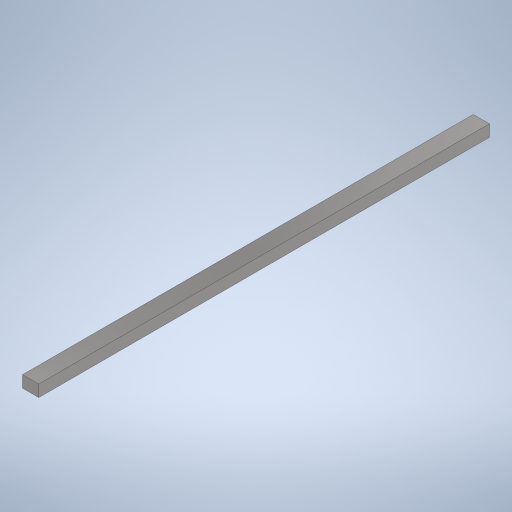
# Autodesk Inventor part: MGN9_rail
Saved by Autodesk Inventor 2024 (Build 280153000, 153)
## iProperties
Created: 2023-08-11
Part Number: MGN9_rail
Material: Generic
Document SubType Name: Modeling
Designer: l1534
Density: 1 g/cm^3
Appearance: Stainless - Brushed
Author: l1534
Autodesk Inventor part; units mm, degrees
ref_plane "YZ Plane" through (0, 0, 0) normal (1, 0, 0) x (0, 1, 0)
ref_plane "XZ Plane" through (0, 0, 0) normal (0, 1, 0) x (-1, 0, 0)
ref_plane "XY Plane" through (0, 0, 0) normal (0, 0, 1) x (1, 0, 0)
sketch "Sketch1" plane through (0, 0, 0) normal (0, 0, 1) x (1, 0, 0)
  line L0 (-4.9415, 4.4682) -> (4.0585, 4.4682)
  line L1 (4.0585, 4.4682) -> (4.0585, -2.0318)
  line L2 (4.0585, -2.0318) -> (-4.9415, -2.0318)
  line L3 (-4.9415, -2.0318) -> (-4.9415, 4.4682)
  point P0 (0, 0)
  dimension "d0" = 9
  dimension "d1" = 6.5
  constraints: 8 end point, 2 parallel, 1 horizontal, 1 perpendicular
  measures "d0" distance of L0.start L0.end
  measures "d1" distance of L0.end L1.end
extrude "Extrusion1" add sketch "Sketch1" along normal blind 250
body "Solid1"
